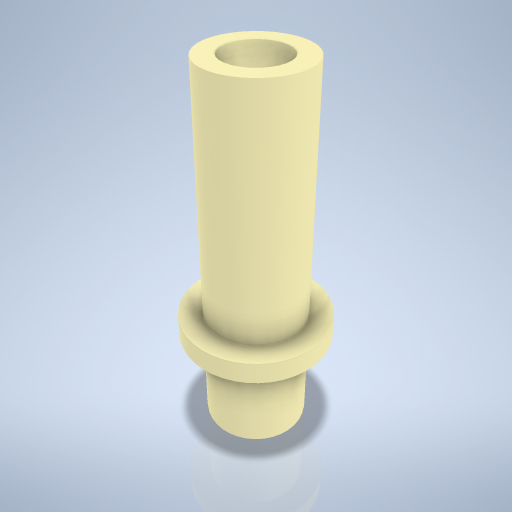
# Autodesk Inventor part: 07
Saved by Autodesk Inventor 2024.2 (Build 282272000, 272)
## iProperties
Created: 2024-05-14
Part Number: 07
Material: Nylon 6/6
Document SubType Name: Modeling
Designer: Fabri
Density: 1.13 g/cm^3
Appearance: Nylon 6
Author: Fabri
Autodesk Inventor part; units mm, degrees
ref_plane "YZ Plane" through (0, 0, 0) normal (1, 0, 0) x (0, 1, 0)
ref_plane "XZ Plane" through (0, 0, 0) normal (0, 1, 0) x (-1, 0, 0)
ref_plane "XY Plane" through (0, 0, 0) normal (0, 0, 1) x (1, 0, 0)
sketch "Skizze1" plane through (0, 0, 0) normal (0, 1, 0) x (-1, 0, 0)
  line L0 (0, 0) -> (3.25, 0)
  line L1 (3.25, 0) -> (3.25, -16)
  line L2 (3.25, -16) -> (4.75, -16)
  line L3 (4.75, -16) -> (4.75, -17.5)
  line L4 (4.75, -17.5) -> (3.25, -17.5)
  line L5 (3.25, -17.5) -> (3.25, -24)
  line L6 (3.25, -24) -> (0, -24)
  line L7 (0, -24) -> (0, 0)
  point P0 (4.75, -16.75)
  dimension "d0" = 6.5
  dimension "d1" = 9.5
  dimension "d2" = 16
  dimension "d3" = 1.5
  dimension "d4" = 6.5
  constraints: 16 end point, 6 perpendicular, 2 point on line, 1 horizontal, 1 midpoint
  measures "d0" diameter of L1 L7
  measures "d1" diameter of point (4.75, -16.75) L7
  measures "d2" distance between parallel lines of L0 L2
  measures "d3" distance between parallel lines of L4 L2
  measures "d4" distance between parallel lines of L4 L6
revolve "Umdrehung1" add sketch "Skizze1" angle 360 about axis through (0, 0, -24) along (0, 0, 1)
sketch "Skizze2" plane through (0, 0, -24) normal (0, 0, -1) x (-1, 0, 0)
  circle A0 centre (0, 0) radius 3.25 projected
  constraints: 1 coincident
hole "Bohrung1" at (0, 0, -24) direction (0, 0, 1) diameter 4 depth 24
